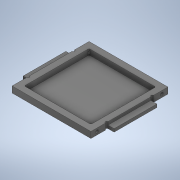
# Autodesk Inventor part: Cockpit_vertical_frame_02
Saved by Autodesk Inventor 2020.4 (Build 244396000, 396)
## iProperties
Created: 2021-04-12
Part Number: Cockpit_vertical_frame_02
Material: アセタール樹脂、黒
Document SubType Name: Modeling
Designer: Masato Kubotera
Density: 1.425 g/cm^3
Appearance: 滑らか - 黒
Mass: 5.96338 g
Surface Area: 41.6737 cm^2
Volume: 4.18483 cm^3
Author: Masato Kubotera
Title: Cockpit_vertical_frame_02
Autodesk Inventor part; units mm, degrees
ref_plane "YZ Plane" through (0, 0, 0) normal (1, 0, 0) x (0, 1, 0)
ref_plane "XZ Plane" through (0, 0, 0) normal (0, 1, 0) x (-1, 0, 0)
ref_plane "XY Plane" through (0, 0, 0) normal (0, 0, 1) x (1, 0, 0)
sketch "スケッチ1" plane through (0, 0, 0) normal (0, 0, 1) x (1, 0, 0)
  line L0 (-32.25, 31.5) -> (-32.25, 19.6)
  line L1 (-37.25, 17.5) -> (-32.25, 17.5)
  line L2 (-37.25, -17.5) -> (-32.25, -17.5)
  arc A0 (-32.25, 17.5) -> (-32.25, 19.6) centre (-32.25, 18.55) ccw
  arc A1 (-32.25, -19.6) -> (-32.25, -17.5) centre (-32.25, -18.55) ccw
  line L3 (-37.25, -17.5) -> (-37.25, 17.5)
  line L4 (-32.25, -19.6) -> (-32.25, -31.5)
  line L5 (-32.25, 31.5) -> (32.25, 31.5)
  line L6 (32.25, -31.5) -> (-32.25, -31.5)
  line L7 (32.25, 31.5) -> (32.25, 19.6)
  line L8 (37.25, 17.5) -> (32.25, 17.5)
  line L9 (37.25, -17.5) -> (32.25, -17.5)
  arc A2 (32.25, 19.6) -> (32.25, 17.5) centre (32.25, 18.55) ccw
  arc A3 (32.25, -17.5) -> (32.25, -19.6) centre (32.25, -18.55) ccw
  line L10 (32.25, -19.6) -> (32.25, -31.5)
  line L11 (37.25, 17.5) -> (37.25, -17.5)
  line L12 (32.25, 17.5) -> (32.25, -17.5)
  line L13 (-32.25, 17.5) -> (-32.25, -17.5)
  line L14 (-32.25, -31.5) -> (32.25, 31.5) construction
  line L15 (-32.25, 31.5) -> (32.25, -31.5) construction
  line L16 (-37.25, 17.5) -> (37.25, -17.5) construction
  line L17 (-37.25, -17.5) -> (37.25, 17.5) construction
  line L18 (-37.25, 0) -> (37.25, 0) construction
  line L19 (0, 31.5) -> (0, -31.5) construction
  line L20 (-27.25, 26.5) -> (27.25, 26.5)
  line L21 (27.25, 26.5) -> (27.25, -26.5)
  line L22 (27.25, -26.5) -> (-27.25, -26.5)
  line L23 (-27.25, -26.5) -> (-27.25, 26.5)
  line L24 (-27.25, 26.5) -> (27.25, -26.5) construction
  line L25 (27.25, 26.5) -> (-27.25, -26.5) construction
  point P0 (0, 0)
  point P1 (0, 0)
  dimension "凸幅" = 35
  dimension "エンドミル逃げ径" = 1.05
  dimension "長さ" = 63
  dimension "凸長" = 5
  dimension "幅" = 64.5
  dimension "エンドミル逃げ径2" = 1.05
  dimension "エンドミル逃げ径3" = 1.05
  dimension "エンドミル逃げ径4" = 1.05
  dimension "凸長2" = 5
  dimension "d71" = 5
  dimension "d72" = 5
  constraints: 52 end point, 9 midpoint, 8 perpendicular, 8 point on circle, 7 point on line, 5 parallel, 4 centre point, 3 collinear, 2 horizontal, 2 vertical, 1 coincident, 1 tangent
  measures "凸幅" distance between parallel lines of L2 L1
  measures "エンドミル逃げ径" radius of A0
  measures "長さ" distance between parallel lines of L6 L5
  measures "凸長" distance between parallel lines of L3 L0
  measures "幅" distance of L0.start L5.end
  measures "エンドミル逃げ径2" radius of A2
  measures "エンドミル逃げ径3" radius of A1
  measures "エンドミル逃げ径4" radius of A3
  measures "凸長2" distance between parallel lines of L12 L11
  measures "d71" distance between parallel lines of L6 L22
  measures "d72" distance between parallel lines of L12 L21
extrude "押し出し1" add sketch "スケッチ1" along normal blind 2.5
extrude "押し出し2" add sketch "スケッチ1" along normal blind 5 contours L5 L7 A2 L12 A3 L10 L6 L4 A1 L13 A0 L0
sketch "スケッチ2" plane through (32.25, 19.6, 0) normal (1, 0, 0) x (0, 0, -1)
  line L0 (0, -51.1) -> (0, -39.2) projected
  line L1 (-2.5, 11.9) -> (-2.5, -51.1) construction
  line L2 (0, -51.1) -> (-5, -51.1) construction
  line L3 (0, 11.9) -> (-5, 11.9) projected
  point P0 (0, -19.6)
  point P1 (-2.5, 6.9)
  point P2 (-2.5, -46.1)
  dimension "d69" = 5
  dimension "d70" = 5
  constraints: 2 end point, 2 midpoint, 2 point on line
  measures "d69" distance of L1.start point (-2.5, 6.9)
  measures "d70" distance of L1.end point (-2.5, -46.1)
hole "穴1" at (32.25, 26.5, 2.5) at (32.25, -26.5, 2.5) direction (-1, 0, 0) diameter 2.459 depth 5 thread size "M3x0.5" class "6H" standard "ISO Metric profile"
sketch "スケッチ3" plane through (-32.25, 19.6, 0) normal (-1, 0, 0) x (0, 0, 1)
  arc A0 (3.7295, 6.9) -> (1.2705, 6.9) centre (2.5, 6.9) ccw projected
  arc A1 (1.2705, -46.1) -> (3.7295, -46.1) centre (2.5, -46.1) ccw projected
  point P0 (2.5, 6.9)
  point P1 (2.5, -46.1)
  constraints: 2 coincident
hole "穴2" at (-32.25, 26.5, 2.5) at (-32.25, -26.5, 2.5) direction (1, 0, 0) diameter 2.459 depth 5 thread size "M3x0.5" class "6H" standard "ISO Metric profile"
fillet "フィレット1" radius 1 12 edges at (-27.25, 26.5, 4.3647) (-27.25, 26.5, 2.5) (-27.25, 26.5, 0.6352) (-27.25, -26.5, 4.3647) (-27.25, -26.5, 2.5) (-27.25, -26.5, 0.6353) (27.25, -26.5, 2.5) (27.25, -26.5, 4.3647) (27.25, -26.5, 0.6352) (27.25, 26.5, 2.5) (27.25, 26.5, 4.3647) (27.25, 26.5, 0.6352)
extrude "押し出し3" add sketch "スケッチ1" along normal blind 0.5 contours L20 L21 L22 L23
equation "\"エンドミル逃げ径2\" = エンドミル逃げ径"
equation "\"エンドミル逃げ径3\" = エンドミル逃げ径"
equation "\"エンドミル逃げ径4\" = エンドミル逃げ径"
equation "\"凸長2\" = 凸長"
equation "\"d70\" = d69"
equation "\"穴長2\" = 穴長"
equation "\"ネジ切り長2\" = ネジ切り長"
equation "\"穴長\" = 5"
equation "\"ネジ切り長\" = 5"
